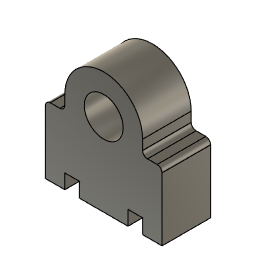
Part 5 (Autodesk Fusion 360 design; units mm, degrees)
Autodesk Fusion 360 part; units mm, degrees
sketch "Sketch1" plane through (0, 0, 0) normal (0, 1, 0) x (1, 0, 0)
  line L0 (-147.5, 45) -> (-147.5, -95)
  line L1 (92.5, -95) -> (92.5, 45)
  line L2 (52.5, 45) -> (52.5, 15)
  line L3 (22.5, 15) -> (22.5, 45)
  line L4 (52.5, 15) -> (22.5, 15)
  line L5 (-107.5, 45) -> (-107.5, 15)
  line L6 (-107.5, 15) -> (-77.5, 15)
  line L7 (-77.5, 15) -> (-77.5, 45)
  line L8 (-107.5, 45) -> (-147.5, 45)
  line L9 (92.5, 45) -> (52.5, 45)
  line L10 (22.5, 45) -> (-77.5, 45)
  line L11 (-107.5, -95) -> (-107.5, -125)
  line L12 (52.5, -125) -> (52.5, -95)
  line L13 (-147.5, -95) -> (-107.5, -95)
  line L14 (52.5, -95) -> (92.5, -95)
  arc A0 (-107.5, -125) -> (52.5, -125) centre (-27.5, -125) ccw
  dimension "d1" = 40
  dimension "d2" = 30
  dimension "d3" = 40
  dimension "d4" = 30
  dimension "d5" = 100
  dimension "d6" = 30
  dimension "d7" = 30
  dimension "d8" = 120
  dimension "d9" = 140
  dimension "d10" = 40
  dimension "d11" = 170
  constraint horizontal L9
  constraint vertical L0
  constraint horizontal L13
  constraint vertical L1
  constraint perpendicular L2 L9
  constraint coincident L3.end L9
  constraint perpendicular L3 L9
  constraint perpendicular L3 L4
  constraint coincident L5.start L9
  constraint perpendicular L5 L9
  constraint perpendicular L5 L6
  constraint perpendicular L7 L9
  constraint collinear L8 L9
  constraint collinear L9 L10
  constraint perpendicular L11 L13
  constraint coincident L12.end L13
  constraint perpendicular L12 L13
  constraint collinear L13 L14
  constraint tangent L11 A0
  constraint tangent L12 A0
  measures "d1" distance of L1.end L2.start
  measures "d2" distance of L2.end L3.start
  measures "d3" distance of L0.start L5.start
  measures "d4" distance of L5.end L6.end
  measures "d5" distance of L3.end L7.end
  measures "d6" distance of L5.start L5.end
  measures "d7" distance of L3.start L3.end
  measures "d8" distance of L0 A0.centre
  measures "d9" distance of L0.start L0.end
  measures "d10" distance of L0.end L11.start
  measures "d11" distance of L10 A0.centre
extrude "Extrude1" add sketch "Sketch1" along normal blind 100
sketch "Sketch2" plane through (0, 0, 0) normal (0, -1, 0) x (1, 0, 0)
  line L0 (-147.5, -45) -> (-107.5, -45)
  line L1 (-107.5, -45) -> (-107.5, -15)
  line L2 (-107.5, -15) -> (-77.5, -15)
  line L3 (-77.5, -15) -> (-77.5, -45)
  line L4 (-77.5, -45) -> (22.5, -45)
  line L5 (22.5, -45) -> (22.5, -15)
  line L6 (22.5, -15) -> (52.5, -15)
  line L7 (52.5, -15) -> (52.5, -45)
  line L8 (52.5, -45) -> (92.5, -45)
  line L9 (92.5, -45) -> (92.5, 95)
  line L10 (92.5, 95) -> (52.5, 95)
  line L11 (52.5, 95) -> (52.5, 125)
  arc A0 (52.5, 125) -> (-107.5, 125) centre (-27.5, 125) ccw
  line L12 (-107.5, 125) -> (-107.5, 95)
  line L13 (-107.5, 95) -> (-147.5, 95)
  line L14 (-147.5, 95) -> (-147.5, -45)
  circle A1 centre (-27.5, 125) radius 40
  dimension "d14" = 80
  constraint concentric A0 A1
  measures "d14" diameter of A1
extrude "Extrude2" cut sketch "Sketch2" against normal blind 100 contours A1
fillet "Fillet1" radius 10 2 edges at (52.5, 50, 95) (-107.5, 50, 95)
fillet "Fillet2" radius 10 2 edges at (92.5, 50, 95) (-147.5, 50, 95)
